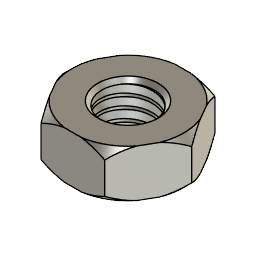
M4_hex_nut (Autodesk Fusion 360 design; units mm, degrees)
part number: 2026-04-25-09-47-30-495
Autodesk Fusion 360 part; units mm, degrees
sketch "Hex Nut Shape" plane through (0, 0, 0) normal (0, 0, 1) x (1, 0, 0)
  line L0 (-2.0207, 3.5) -> (-4.0415, 0)
  line L1 (-4.0415, 0) -> (-2.0207, -3.5)
  line L2 (-2.0207, -3.5) -> (2.0207, -3.5)
  line L3 (2.0207, -3.5) -> (4.0415, 0)
  line L4 (4.0415, 0) -> (2.0207, 3.5)
  line L5 (2.0207, 3.5) -> (-2.0207, 3.5)
  dimension "d3" = 7
  measures "d3" distance of L2 L5
extrude "Extrude1" add sketch "Hex Nut Shape" along normal blind 3
sketch "Chamfer Outline" plane through (0, 0, 0) normal (0, 1, 0) x (1, 0, 0)
  line L0 (2.0207, 0) -> (4.0415, 0)
  line L1 (4.0415, 0) -> (4.0415, -3)
  line L2 (4.0415, -3) -> (2.0207, -3)
  line L3 (2.0207, -3) -> (2.0207, 0)
  line L4 (-2.0207, 0) -> (2.0207, 0)
  line L5 (2.0207, 0) -> (2.0207, -3)
  line L6 (2.0207, -3) -> (-2.0207, -3)
  line L7 (-2.0207, -3) -> (-2.0207, 0)
  line L8 (-4.0415, 0) -> (-2.0207, 0)
  line L9 (-2.0207, 0) -> (-2.0207, -3)
  line L10 (-2.0207, -3) -> (-4.0415, -3)
  line L11 (-4.0415, -3) -> (-4.0415, 0)
  line L12 (4.0415, -3) -> (3.5415, -3)
  line L13 (4.0415, -3) -> (4.0415, -2.5)
  line L14 (4.0415, 0) -> (4.0415, -0.5)
  line L15 (4.0415, 0) -> (3.5415, 0)
  line L16 (3.5415, -3) -> (4.0415, -2.5)
  line L17 (4.0415, -0.5) -> (3.5415, 0)
  dimension "d11" = 0.5
  dimension "d12" = 0.5
  dimension "d13" = 0.5
  dimension "d14" = 0.5
  constraint coincident L1.end L2.start
  constraint perpendicular L1 L12
  constraint coincident L1 L13.end
  constraint coincident L0.end L1.start
  constraint perpendicular L2 L14
  constraint perpendicular L14 L15
  measures "d11" distance of L1.end L12.end
  measures "d12" distance of L1.end L13.end
  measures "d13" distance of L0.end L14.end
  measures "d14" distance of L0.end L15.end
revolve "Revolve1" cut sketch "Chamfer Outline" angle 360 about axis through (0, 0, 1.75) along (0, 0, 1) contours L0 L1 L14 L15 L17 | L1 L2 L12 L13 L16
hole "Hole1" at (0, 0, 3) direction (0, 0, -1) diameter 4 end through all
chamfer "Chamfer1" distance 0.25 angle 45 2 edges at (-1.8647, 0.7232, 3) (-1.8647, -0.7232, 0)
thread "Thread2" "ISO Metric profile 4.0 M4x0.7 M4x0.7 6H" major diameter 4.1095 minor diameter 3.332 pitch 0.7 angle 60 modelled right hand crest width 0.193 on face at (0.1991, -1.9901, 1.9167) crest through (1.666, 0, 2.575)
equation "width_across_flats = 7 mm" comment "An M4 hex nut has a width across the flats of 7 mm."
equation "thickness = 3 mm" comment "An M4 hex nut has a thickness of 3 mm."
equation "d3 = width_across_flats"
equation "d4 = thickness"
equation "chamfer_side_length = 0.5 mm" comment "Chamfer on the outside top and bottom of the hex nut."
equation "d11 = chamfer_side_length"
equation "d12 = chamfer_side_length"
equation "d13 = chamfer_side_length"
equation "d14 = chamfer_side_length"
equation "d16 = hole_diameter"
equation "hole_diameter = 4 mm" comment "An M4 hex nut has a hole diameter of 4 mm."
equation "hole_chamfer = 0.25 mm" comment "Chamfer on the inside of the hex nut thread hole."
equation "d20 = hole_chamfer"
named bodies: "M4 Hex Nut"
